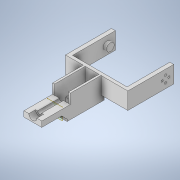
# Autodesk Inventor part: Joint2
Saved by Autodesk Inventor 2022 (Build 260153000, 153)
## iProperties
Created: 2022-02-25
Part Number: Joint2
Material: Generic
Document SubType Name: Modeling
Designer: Mlees
Density: 1 g/cm^3
Appearance: Default
Author: Mlees
Autodesk Inventor part; units mm, degrees
ref_plane "YZ Plane" through (0, 0, 0) normal (1, 0, 0) x (0, 1, 0)
ref_plane "XZ Plane" through (0, 0, 0) normal (0, 1, 0) x (-1, 0, 0)
ref_plane "XY Plane" through (0, 0, 0) normal (0, 0, 1) x (1, 0, 0)
sketch "Sketch1" plane through (0, 0, 0) normal (0, 1, 0) x (-1, 0, 0)
  line L0 (0, 0) -> (0, -81.8644)
  line L1 (4.678, -40.9322) -> (4.678, 5.8475)
  line L2 (4.678, -40.9322) -> (4.678, -87.7119)
  line L3 (4.678, 5.8475) -> (-64.322, 5.8475)
  line L4 (-64.322, 5.8475) -> (-64.322, 0)
  line L5 (-64.322, 0) -> (0, 0)
  line L6 (0, -81.8644) -> (-64.322, -81.8644)
  line L7 (-64.322, -81.8644) -> (-64.322, -87.7119)
  line L8 (-64.322, -87.7119) -> (4.678, -87.7119)
  dimension "d4" = 69
  constraints: 18 end point, 4 perpendicular, 2 horizontal, 2 vertical
  measures "d4" distance of L1.end L3.end
extrude "Extrusion1" add sketch "Sketch1" along normal blind 25.4
sketch "Sketch2" plane through (-4.678, 0, -87.7119) normal (-1, 0, 0) x (0, 0, 1)
  line L0 (87.7119, 25.4) -> (5.8475, 25.4) projected
  line L1 (87.7119, 0) -> (5.8475, 0) projected
  line L2 (40, -8.93) -> (50.35, -8.93)
  line L3 (50.35, -8.93) -> (53.35, -8.93)
  line L4 (40, -8.93) -> (29.65, -8.93)
  line L5 (29.65, -8.93) -> (26.65, -8.93)
  line L6 (53.35, -8.93) -> (53.35, 25.4)
  line L7 (26.65, -8.93) -> (26.65, 25.4)
  line L8 (26.65, 25.4) -> (53.35, 25.4)
  dimension "d19" = 3
  dimension "d20" = 10.35
  dimension "d26" = 34.33
  constraints: 14 end point, 3 horizontal, 3 point on line, 2 perpendicular, 1 collinear
  measures "d19" distance of L2.end L3.end
  measures "d20" distance of L2.start L4.end
  measures "d26" distance between parallel lines of L2 L0
extrude "Extrusion2" add sketch "Sketch2" along normal blind 46
sketch "Sketch3" plane through (0, 25.4, 0) normal (0, 1, 0) x (1, 0, 0)
  line L0 (-50.678, 34.3619) -> (-50.678, 61.0619) projected
  line L1 (-50.678, 47.7119) -> (-50.678, 58.0619)
  line L2 (-50.678, 47.7119) -> (-50.678, 37.3619)
  line L3 (-50.678, 58.0619) -> (-4.678, 58.0619)
  line L4 (-4.678, 61.0619) -> (-4.678, 34.3619) projected
  line L5 (-4.678, 58.0619) -> (-4.678, 37.3619)
  line L6 (-4.678, 37.3619) -> (-50.678, 37.3619)
  point P0 (0, 0)
  dimension "d24" = 10.35
  dimension "d25" = 10.35
  constraints: 10 end point, 4 point on line, 1 horizontal, 1 midpoint, 1 perpendicular
  measures "d24" distance of L1.start L1.end
  measures "d25" distance of L1.start L2.end
extrude "Extrusion3" cut sketch "Sketch3" against normal blind 31.33
sketch "Sketch4" plane through (0, -5.93, 0) normal (0, 1, 0) x (1, 0, 0)
  line L0 (-50.678, 61.0619) -> (-50.678, 34.3619) projected
  line L1 (-33.878, 47.7119) -> (-33.878, 58.0619)
  line L2 (-50.678, 58.0619) -> (-4.678, 58.0619) projected
  line L3 (-33.878, 58.0619) -> (-26.878, 58.0619)
  line L4 (-26.878, 58.0619) -> (-26.878, 37.3619)
  line L5 (-4.678, 37.3619) -> (-50.678, 37.3619) projected
  line L6 (-26.878, 37.3619) -> (-33.878, 37.3619)
  line L7 (-33.878, 37.3619) -> (-33.878, 47.7119)
  point P0 (0, 0)
  dimension "d30" = 7
  constraints: 10 end point, 4 perpendicular, 3 point on line, 1 vertical
  measures "d30" distance of L1.end L3.end
extrude "Extrusion4" add sketch "Sketch4" along normal blind 6 contours L2 L4 L5 L7 L1
sketch "Sketch5" plane through (-33.878, -5.93, -58.0619) normal (-1, 0, 0) x (0, 0, 1)
  line L0 (20.7, 0) -> (20.7, 5.93) projected
  line L1 (0, 6) -> (0, 0) projected
  circle A0 centre (5.35, 3) radius 1
  circle A1 centre (15.35, 2.965) radius 1.035
  point P0 (58.0619, 5.93)
  dimension "d35" = 2
  constraints: 2 centre point
  measures "d35" diameter of A0
extrude "Extrusion5" cut sketch "Sketch5" against normal through all
sketch "Sketch6" plane through (-4.678, -8.93, -34.3619) normal (0, 0, 1) x (1, 0, 0)
  line L0 (-29.2, 3) -> (-46, 3) projected
  line L1 (0, 0) -> (-46, 0) projected
  line L2 (-46, 0) -> (-51, 0)
  line L3 (-51, 0) -> (-51, 3)
  line L4 (-59, 11.315) -> (-51, 3)
  line L5 (-51, 19.63) -> (-46, 19.63)
  line L6 (-46, 0) -> (-46, 34.33) projected
  line L7 (69, 8.93) -> (69, 34.33) projected
  line L8 (-59, 11.315) -> (-89, 11.315)
  line L9 (-89, 11.315) -> (-89, 19.63)
  line L10 (-89, 19.63) -> (-51, 19.63)
  point P0 (4.678, 8.93)
  dimension "d41" = 5
  dimension "d42" = 16.63
  dimension "d46" = 30
  constraints: 14 end point, 3 horizontal, 3 perpendicular, 2 point on line
  measures "d41" distance of L1.end L2.end
  measures "d42" distance of L3.end L5.start
  measures "d46" distance of L4.start L8.end
extrude "Extrusion6" add sketch "Sketch6" against normal up to surface (26.7 mm away)
sketch "Sketch7" plane through (-93.678, 2.385, -34.3619) normal (-1, 0, 0) x (0, 0, 1)
  line L0 (-3, 8.315) -> (-23.7, 8.315) projected
  circle A0 centre (-13.35, 8.315) radius 3
  point P0 (34.3619, -2.385)
  point P1 (-16.35, 8.315)
  point P2 (-10.35, 8.315)
  dimension "d49" = 6
  constraints: 1 centre point, 1 midpoint
  measures "d49" diameter of A0
extrude "Extrusion7" cut sketch "Sketch7" against normal up to surface (43 mm away) contours A0 L0 picked at (-13.9181, 7.492)
sketch "Sketch8" plane through (-93.678, 2.385, -34.3619) normal (-1, 0, 0) x (0, 0, 1)
  arc A0 (-16.35, 8.315) -> (-10.35, 8.315) centre (-13.35, 8.315) ccw projected
  circle A1 centre (-13.35, 8.315) radius 6
  point P0 (34.3619, -2.385)
  dimension "d52" = 12
  constraints: 1 centre point, 1 coincident
  measures "d52" diameter of A1
extrude "Extrusion8" cut sketch "Sketch8" against normal blind 10
sketch "Sketch9" plane through (-55.678, -8.93, -34.3619) normal (-1, 0, 0) x (0, 0, 1)
  circle A0 centre (-8.35, 5.965) radius 3.5
  circle A1 centre (-18.35, 6) radius 1 projected
  circle A2 centre (-18.35, 6) radius 3.5
  point P0 (34.3619, 8.93)
  dimension "d55" = 7
  dimension "d56" = 7
  constraints: 2 centre point, 2 coincident
  measures "d55" diameter of A0
  measures "d56" diameter of A2
extrude "Extrusion9" cut sketch "Sketch9" along normal blind 7 and the other way blind 5 contours A0 | A1 | A2
sketch "Sketch10" plane through (-4.678, 0, -87.7119) normal (1, 0, 0) x (0, 0, -1)
  line L0 (-53.35, -5.93) -> (-53.35, -8.93) projected
  line L1 (-50.35, 10.7) -> (-50.35, -5.93) projected
  line L2 (-53.35, -8.93) -> (-50.35, -8.93)
  line L3 (-50.35, -5.93) -> (-50.35, 0)
  line L4 (-50.35, 0) -> (-53.35, 0)
  line L5 (-53.35, 0) -> (-53.35, -8.93)
  line L6 (-26.65, -5.93) -> (-26.65, -8.93) projected
  line L7 (-29.65, -5.93) -> (-29.65, 10.7) projected
  line L8 (-26.65, -8.93) -> (-29.65, -8.93)
  line L9 (-29.65, -5.93) -> (-29.65, 0)
  line L10 (-29.65, 0) -> (-26.65, 0)
  line L11 (-26.65, 0) -> (-26.65, -8.93)
  line L12 (-29.65, -8.93) -> (-50.35, -8.93)
  line L13 (-50.35, 0) -> (-29.65, 0)
  line L14 (-29.65, 0) -> (-29.65, -5.93)
  line L15 (-50.35, -5.93) -> (-50.35, 0)
  point P0 (-87.7119, 0)
  constraints: 24 end point, 5 parallel, 3 horizontal, 3 perpendicular, 3 point on line
extrude "Extrusion10" add sketch "Sketch10" along normal up to surface (4.678 mm away)
sketch "Sketch13" plane through (0, 0, -81.8644) normal (0, 0, 1) x (1, 0, 0)
  line L0 (64.322, 0) -> (64.322, 25.4) projected
  circle A0 centre (51.822, 12.7) radius 5.75
  point P0 (0, 0)
  dimension "d76" = 11.5
  constraints: 1 centre point
  measures "d76" diameter of A0
extrude "Extrusion13" add sketch "Sketch13" along normal blind 5
sketch "Sketch14" plane through (-4.678, 0, 5.8475) normal (0, 0, 1) x (1, 0, 0)
  line L0 (69, 0) -> (69, 25.4) projected
  circle A0 centre (56.5, 12.7) radius 5.75 projected
  circle A1 centre (56.5, 17.7) radius 1.5
  circle A2 centre (51.5, 12.7) radius 1.5
  circle A3 centre (56.5, 7.7) radius 1.5
  circle A4 centre (61.5, 12.7) radius 1.5
  point P0 (4.678, 0)
  dimension "d80" = 3
  dimension "d83" = 360
  constraints: 4 centre point, 1 coincident, 9 other
  measures "d80" diameter of A1
extrude "Extrusion14" cut sketch "Sketch14" against normal up to surface (5.8475 mm away) contours A0 A4 | A0 A4 | A1 A0 | A0 A1 | A3 A0 | A0 A3 | A2 A0 | A0 A2
ref_plane "Work Plane6" through (-60.678, -5.93, -58.0619) normal (1, 0, 0) x (0, 0, -1)
body "Solid1"
